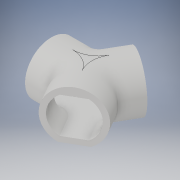
# Autodesk Inventor part: 3 way corridor
Saved by Autodesk Inventor 2017 (Build 210142000, 142)
## iProperties
Created: 2018-03-04
Part Number: 3 way corridor
Material: Generic
Document SubType Name: Modeling
Designer: Braxton
Density: 1 g/cm^3
Appearance: Default
Author: Braxton
Autodesk Inventor part; units mm, degrees
ref_plane "YZ Plane" through (0, 0, 0) normal (1, 0, 0) x (0, 1, 0)
ref_plane "XZ Plane" through (0, 0, 0) normal (0, 1, 0) x (-1, 0, 0)
ref_plane "XY Plane" through (0, 0, 0) normal (0, 0, 1) x (1, 0, 0)
sketch "Sketch1" plane through (0, 0, 0) normal (1, 0, 0) x (0, 1, 0)
  line L0 (-84.666667, 50.8) -> (-84.666667, -50.8)
  arc A0 (-110.066667, -57.405887) -> (-110.066667, 57.405887) centre (0, 0) ccw
  arc A1 (84.666667, 50.8) -> (-84.666667, 50.8) centre (0, 0) ccw
  arc A2 (-84.666667, -50.8) -> (84.666667, -50.8) centre (0, 0) ccw
  line L1 (-110.066667, 57.405887) -> (-110.066667, -57.405887)
  line L2 (84.666667, 8.995833) -> (84.666667, -8.995833) construction
  arc A3 (84.666667, 8.995833) -> (86.254167, 7.408333) centre (86.254167, 8.995833) ccw
  line L3 (87.841667, -7.408333) -> (86.254167, -7.408333)
  line L4 (84.666667, 0) -> (87.841667, 0) construction
  line L5 (87.841667, 7.408333) -> (86.254167, 7.408333)
  arc A4 (86.254167, -7.408333) -> (84.666667, -8.995833) centre (86.254167, -8.995833) ccw
  line L6 (84.666667, 50.8) -> (84.666667, 8.995833)
  line L7 (84.666667, -8.995833) -> (84.666667, -50.8)
  line L8 (84.666667, 4.084376) -> (84.666667, 0)
  line L9 (87.841667, 6.35) -> (87.841667, 0)
  line L10 (87.841667, 6.35) -> (86.913229, 6.35)
  arc A5 (86.913229, 6.35) -> (84.666667, 4.084376) centre (86.932372, 4.084376) ccw
  line L11 (84.666667, 0) -> (87.841667, 0) construction
  line L12 (84.666667, -4.084376) -> (84.666667, 0)
  line L13 (87.841667, -6.35) -> (87.841667, 0)
  arc A6 (84.666667, -4.084376) -> (86.913229, -6.35) centre (86.932372, -4.084376) ccw
  line L14 (87.841667, -6.35) -> (86.913229, -6.35)
  line L15 (87.841667, 6.35) -> (87.841667, 7.408333)
  line L16 (87.841667, -6.35) -> (87.841667, -7.408333)
  dimension "d11" = 101.6
  dimension "d14" = 248.2749
  dimension "d46" = 25.4
  dimension "d51" = 14.81667
  dimension "d52" = 1.5875
  dimension "d53" = 1.5875
  dimension "d55" = 1.5875
  dimension "d61" = 6.35
  dimension "d64" = 2.26571
  dimension "d65" = 2.24656
  dimension "d74" = 84.66667
  constraints: 34 end point, 14 point on circle, 7 centre point, 7 symmetric about line, 6 vertical, 3 horizontal, 2 coincident, 2 parallel, 2 perpendicular, 2 tangent, 1 collinear, 1 midpoint, 2 other
  measures "d11" distance of L6.start L7.end
  measures "d14" diameter of A0
  measures "d46" distance between parallel lines of L0 L1
  measures "d51" distance of L5.start L3.start
  measures "d52" distance from line of L2.end L3
  measures "d53" radius of A4
  measures "d55" distance of L5.start L5.end
  measures "d61" distance of L4.end L9.start
  measures "d64" radius of A5
  measures "d65" horizontal distance of L8.start L10.end
  measures "d74" distance from line of point (0, 0) L6
sketch "Sketch1 outline for corridor" plane through (0, 0, 0) normal (1, 0, 0) x (0, 1, 0)
  arc A0 (-110.066667, 57.405887) -> (-110.066667, -57.405887) centre (0, 0) cw
  line L0 (-110.066667, -57.405887) -> (-110.066667, 57.405887)
  line L1 (87.841667, -6.35) -> (87.841667, 0)
  line L2 (87.841667, 0) -> (87.841667, 6.35)
  line L3 (87.841667, 6.35) -> (87.841667, 7.408333)
  line L4 (87.841667, 7.408333) -> (86.254167, 7.408333)
  arc A1 (86.254167, 7.408333) -> (84.666667, 8.995833) centre (86.254167, 8.995833) cw
  line L5 (84.666667, 8.995833) -> (84.666667, 50.8)
  arc A2 (84.666667, 50.8) -> (-84.666667, 50.8) centre (0, 0) ccw
  line L6 (-84.666667, 50.8) -> (-84.666667, -50.8)
  arc A3 (-84.666667, -50.8) -> (84.666667, -50.8) centre (0, 0) ccw
  line L7 (84.666667, -50.8) -> (84.666667, -8.995833)
  arc A4 (84.666667, -8.995833) -> (86.254167, -7.408333) centre (86.254167, -8.995833) cw
  line L8 (86.254167, -7.408333) -> (87.841667, -7.408333)
  line L9 (87.841667, -7.408333) -> (87.841667, -6.35)
extrude "corridor" add sketch "Sketch1 outline for corridor" along normal blind 101.6
sketch "Sketch1 outline for light" plane through (0, 0, 0) normal (1, 0, 0) x (0, 1, 0)
  line L0 (87.841667, -6.35) -> (87.841667, 0)
  line L1 (86.913229, -6.35) -> (87.841667, -6.35)
  arc A0 (84.666667, -4.084376) -> (86.913229, -6.35) centre (86.932372, -4.084376) ccw
  line L2 (84.666667, 0) -> (84.666667, -4.084376)
  line L3 (84.666667, 4.084376) -> (84.666667, 0)
  arc A1 (86.913229, 6.35) -> (84.666667, 4.084376) centre (86.932372, 4.084376) ccw
  line L4 (87.841667, 6.35) -> (86.913229, 6.35)
  line L5 (87.841667, 0) -> (87.841667, 6.35)
extrude "light" add sketch "Sketch1 outline for light" along normal up to surface (101.6 mm away) separate body
sketch "found rotaion axis" plane through (0, 0, 0) normal (0, 1, 0) x (-1, 0, 0)
  line L0 (-101.6, 124.137452) -> (-101.6, -124.137452)
  line L1 (-101.6, -124.137452) -> (-101.6, 124.137452)
  line L2 (-101.6, 0) -> (-173.270792, 0)
  point P0 (0, 0)
  dimension "d15" = 71.67079
  constraints: 4 end point, 1 horizontal, 1 midpoint, 1 vertical
  measures "d15" distance of L2.start L2.end
pattern_circular "other corridors" count 3 over 360 about axis through (173.270792, 0, 0) along (0, 1, 0) of "corridor", "light" bodies 1
sketch "Sketch5" plane through (101.6, 0, 0) normal (1, 0, 0) x (0, 0, -1)
  arc A0 (50.8, -84.666667) -> (50.8, 84.666667) centre (0, 0) ccw
  arc A1 (0, -124.137452) -> (0, 124.137452) centre (0, 0) ccw
  line L0 (50.8, 84.666667) -> (8.995833, 84.666667)
  line L1 (50.8, -84.666667) -> (0, -84.666667)
  line L2 (0, 124.137452) -> (0, 87.841667)
  line L3 (0, -84.666667) -> (0, -124.137452)
  line L4 (-7.408333, 87.841667) -> (7.408333, 87.841667)
  line L5 (7.408333, 87.841667) -> (7.408333, 86.254167)
  arc A2 (7.408333, 86.254167) -> (8.995833, 84.666667) centre (8.995833, 86.254167) ccw
  arc A3 (7.408333, 86.254167) -> (8.995833, 84.666667) centre (8.995833, 86.254167) ccw
  line L6 (-6.35, 87.841667) -> (-6.35, 86.913229)
  line L7 (0, 87.841667) -> (-6.35, 87.841667)
  arc A4 (-6.35, 86.913229) -> (-4.084376, 84.666667) centre (-4.084376, 86.932372) ccw
  line L8 (-6.35, 87.841667) -> (-6.35, 86.913229)
  arc A5 (4.084376, 84.666667) -> (6.35, 86.913229) centre (4.084376, 86.932372) ccw
  line L9 (-4.084376, 84.666667) -> (4.084376, 84.666667)
  line L10 (6.35, 86.913229) -> (6.357845, 87.841667)
  line L11 (0, 87.841667) -> (6.357845, 87.841667)
  line L12 (7.408333, 87.841667) -> (-7.408333, 87.841667)
  line L13 (6.357845, 87.841667) -> (7.408333, 87.841667)
  line L14 (-4.084376, 84.666667) -> (4.084376, 84.666667)
  arc A6 (-6.35, 86.913229) -> (-4.084376, 84.666667) centre (-4.103357, 86.913229) ccw
  arc A7 (4.084376, 84.666667) -> (6.35, 86.913229) centre (4.084376, 86.932372) ccw
  point P0 (6.35, 87.841667)
  constraints: 22 end point, 11 point on circle, 5 centre point, 4 tangent, 2 coincident, 2 collinear, 2 horizontal, 2 point on line, 2 vertical, 1 midpoint, 1 perpendicular
sketch "Sketch4" plane through (0, 0, 0) normal (0, 1, 0) x (-1, 0, 0)
  line L0 (0, -98.737452) -> (-101.6, -98.737452)
  line L1 (-174.397046, -199.425634) -> (-123.597046, -111.437453)
  line L2 (-101.6, -98.737452) -> (0, -98.737452)
  line L3 (0, -124.137452) -> (0, 124.137452)
  line L4 (-123.597046, -111.437453) -> (-174.397046, -199.425634)
  line L5 (-367.412375, -87.988182) -> (-152.400001, -212.125634)
  line L6 (-345.41533, -100.688182) -> (-294.61533, -12.700001)
  line L7 (-345.41533, -100.688182) -> (-294.61533, -12.700001)
  line L8 (-345.41533, 100.688182) -> (-294.61533, 12.700001)
  line L9 (-294.615329, 12.7) -> (-312.526979, 43.723888)
  line L10 (-174.397046, 199.425634) -> (-123.597046, 111.437453)
  line L11 (-123.597046, 111.437453) -> (-165.112098, 87.468727)
  line L12 (-187.474467, 222.076391) -> (-123.597046, 111.437453)
  line L13 (0, 98.737452) -> (-101.6, 98.737452)
  line L14 (-101.600001, 98.737452) -> (0, 98.737452)
  line L15 (-101.600001, -124.137453) -> (-316.612375, -0.000001)
  arc A0 (-101.600001, -98.737452) -> (-123.597047, -111.437452) centre (-101.600001, -124.137453) ccw
  arc A1 (-294.61533, -12.700001) -> (-294.615329, 12.7) centre (-316.612375, -0.000001) ccw
  line L16 (-316.612376, 0) -> (-101.600001, 124.137453)
  arc A2 (-123.597046, 111.437453) -> (-101.600001, 98.737452) centre (-101.600001, 124.137453) ccw
  point P0 (0, 0)
  point P1 (-316.612375, -0.000001)
  point P2 (-244.941584, 103.912102)
  point P3 (-277.182894, 71.670792)
  constraints: 13 end point, 8 point on circle, 8 point on line, 3 centre point, 3 perpendicular, 1 coincident, 5 other
sketch "Sketch5 outline for curve edjes" plane through (101.6, 0, 0) normal (1, 0, 0) x (0, 0, -1)
  arc A0 (0, -124.137452) -> (0, 124.137452) centre (0, 0) ccw
  line L0 (0, -84.666667) -> (0, -124.137452)
  line L1 (50.8, -84.666667) -> (0, -84.666667)
  arc A1 (50.8, 84.666667) -> (50.8, -84.666667) centre (0, 0) cw
  line L2 (8.995833, 84.666667) -> (50.8, 84.666667)
  arc A2 (7.408333, 86.254167) -> (8.995833, 84.666667) centre (8.995833, 86.254167) ccw
  line L3 (7.408333, 87.841667) -> (7.408333, 86.254167)
  line L4 (6.357845, 87.841667) -> (7.408333, 87.841667)
  line L5 (0, 87.841667) -> (6.357845, 87.841667)
  line L6 (0, 124.137452) -> (0, 87.841667)
sweep "curve edjes" add profiles "Sketch5 outline for curve edjes" path "Sketch4" bodies 1 path curves A0
sketch "Sketch5 outline for light curve" plane through (101.6, 0, 0) normal (1, 0, 0) x (0, 0, -1)
  line L0 (0, 87.841667) -> (-6.35, 87.841667)
  line L1 (6.357845, 87.841667) -> (0, 87.841667)
  line L2 (6.35, 86.913229) -> (6.357845, 87.841667)
  arc A0 (4.084376, 84.666667) -> (6.35, 86.913229) centre (4.084376, 86.932372) ccw
  line L3 (-4.084376, 84.666667) -> (4.084376, 84.666667)
  arc A1 (-6.35, 86.913229) -> (-4.084376, 84.666667) centre (-4.084376, 86.932372) ccw
  line L4 (-6.35, 87.841667) -> (-6.35, 86.913229)
sweep "light curve" add profiles "Sketch5 outline for light curve" path "Sketch4" separate body path curves A0
pattern_circular "repeat curve edjes" count 3 over 360 about axis through (173.270792, 0, 0) along (0, 1, 0) of "curve edjes", "light curve" bodies 1
sketch "Sketch9" plane through (101.6, 87.841667, 6.35) normal (0, 1, 0) x (1, 0, 0)
  arc A0 (107.506188, -55.718727) -> (0, 6.35) centre (0, -117.787452) ccw
  arc A1 (107.506188, -55.718727) -> (0, 6.35) centre (0, -117.787453) ccw
  arc A2 (107.506188, 68.418725) -> (107.506188, -55.718727) centre (215.012375, 6.349999) ccw
  arc A3 (107.506188, 68.418725) -> (107.506188, -55.718727) centre (215.012373, 6.349999) ccw
  arc A4 (0, 6.35) -> (107.506188, 68.418725) centre (0.000005, 130.487446) ccw
  point P0 (-101.6, 6.35)
  constraints: 6 point on circle, 3 centre point, 1 equal radius
sketch "Sketch9 outline for top hole fill in" plane through (101.6, 87.841667, 6.35) normal (0, 1, 0) x (1, 0, 0)
  arc A0 (107.506188, 68.418725) -> (0, 6.35) centre (0.000001, 130.487453) cw
  arc A1 (107.506188, -55.718727) -> (107.506188, 68.418725) centre (215.012371, 6.349999) cw
  arc A2 (0, 6.35) -> (107.506188, -55.718727) centre (0.000002, -117.787451) cw
extrude "top hole fill in" add sketch "Sketch9 outline for top hole fill in" along normal blind 36.295785 bodies 3
sketch "Sketch7" plane through (0, -84.666667, 50.8) normal (0, 1, 0) x (1, 0, 0)
  arc A0 (209.106188, -11.268727) -> (101.6, 50.8) centre (101.6, -73.337452) ccw
  arc A1 (209.106188, -11.268727) -> (101.6, 50.8) centre (101.6, -73.337452) ccw
  arc A2 (101.6, 50.8) -> (209.106188, 112.868725) centre (101.600001, 174.937453) ccw
  line L0 (316.612375, 50.800001) -> (209.106188, -11.268727)
  arc A3 (209.106188, 112.868725) -> (209.106188, -11.268727) centre (316.612375, 50.799999) ccw
  arc A4 (209.106188, 112.868725) -> (209.106188, -11.268727) centre (316.612375, 50.799999) ccw
  line L1 (209.106188, 112.868725) -> (316.612375, 50.800001)
  arc A5 (101.6, 50.8) -> (209.106188, 112.868725) centre (101.600001, 174.937453) ccw
  point P0 (173.270792, 50.8)
  constraints: 6 point on circle, 3 centre point, 3 concentric
sketch "Sketch7 outline for bottom hole fill up" plane through (0, -84.666667, 50.8) normal (0, 1, 0) x (1, 0, 0)
  arc A0 (101.6, 50.8) -> (209.106188, -11.268727) centre (101.600002, -73.337451) cw
  arc A1 (209.106188, 112.868725) -> (101.6, 50.8) centre (101.600001, 174.937453) cw
  arc A2 (209.106188, -11.268727) -> (209.106188, 112.868725) centre (316.612371, 50.799999) cw
extrude "bottom hole fill up" add sketch "Sketch7 outline for bottom hole fill up" against normal blind 39.470785 bodies 1
equation "\"d52\" = 0.5 * d54"
equation "\"d54\" = 3.175"
body "Solid1"
body "Solid2"
body "Solid3"
